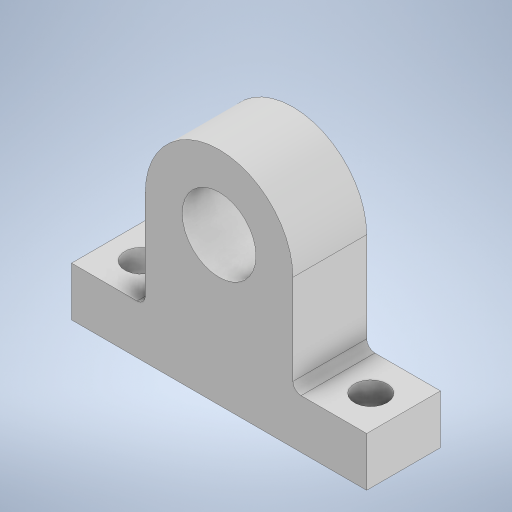
# Autodesk Inventor part: HUDSON 1-04-REAR DRAWBAR BEAM BRACKET
Saved by Autodesk Inventor 2024.2 (Build 282272000, 272)
## iProperties
Created: 2024-09-30
Part Number: HUDSON 1-04-REAR DRAWBAR BEAM BRACKET
Material: Generic
Document SubType Name: Modeling
Designer: Jimena Brenes
Density: 1 g/cm^3
Appearance: Default
Author: Jimena Brenes
Autodesk Inventor part; units mm, degrees
ref_plane "YZ Plane" through (0, 0, 0) normal (1, 0, 0) x (0, 1, 0)
ref_plane "XZ Plane" through (0, 0, 0) normal (0, 1, 0) x (-1, 0, 0)
ref_plane "XY Plane" through (0, 0, 0) normal (0, 0, 1) x (1, 0, 0)
sketch "Sketch1" plane through (0, 0, 0) normal (0, 0, 1) x (1, 0, 0)
  circle A0 centre (0, 0) radius 4.5
  arc A1 (9, 0) -> (-9, 0) centre (0, 0) ccw
  line L0 (0, 0) -> (0, -47) construction
  line L1 (0, -18) -> (-18, -18)
  line L2 (0, -18) -> (18, -18)
  line L3 (18, -18) -> (18, -12)
  line L4 (18, -12) -> (10, -12)
  line L5 (9, -11) -> (9, 0)
  line L6 (-18, -18) -> (-18, -12)
  line L7 (-18, -12) -> (-10, -12)
  line L8 (-9, -11) -> (-9, 0)
  arc A2 (-10, -12) -> (-9, -11) centre (-10, -11) ccw
  arc A3 (9, -11) -> (10, -12) centre (10, -11) ccw
  dimension "d0" = 9
  dimension "d1" = 18
  dimension "d6" = 6
  dimension "d7" = 6
  dimension "d9" = 18
  dimension "d10" = 2
  dimension "d11" = 2
  dimension "d12" = 9
  dimension "d13" = 9
  dimension "d14" = 36
  dimension "d15" = 18
  constraints: 18 end point, 6 point on circle, 5 perpendicular, 4 centre point, 4 tangent, 2 coincident, 2 horizontal, 2 vertical, 1 point on line
  measures "d0" diameter of A0
  measures "d1" diameter of A1
  measures "d6" distance between parallel lines of L2 L4
  measures "d7" distance of L1.end L6.end
  measures "d9" distance from line of L1 point (0, 0)
  measures "d10" diameter of A2
  measures "d11" diameter of A3
  measures "d12" distance from line of L8 L6.end
  measures "d13" distance from line of L5 L3.end
  measures "d14" distance between parallel lines of L3 L6
  measures "d15" distance of L1.start L2.end
extrude "Extrusion1" add sketch "Sketch1" against normal blind 9 contours A0 | L5 A3 L4 L3 L2 L1 L6 L7 A2 L8 A1
hole "Hole1" at (0, 0, 0) direction (0, 0, -1) diameter 9 end through all
sketch "Sketch2" plane through (-18, -12, 0) normal (0, 1, 0) x (1, 0, 0)
  circle A0 centre (4, 4.5) radius 2
  circle A1 centre (32, 4.5) radius 2
  line L0 (8, 0) -> (0, 0) projected
  line L1 (0, 0) -> (0, 9) projected
  line L2 (36, 0) -> (28, 0) projected
  line L3 (36, 0) -> (36, 9) projected
  point P0 (18, 0)
  dimension "d25" = 4
  dimension "d26" = 4
  dimension "d27" = 4.5
  dimension "d28" = 4
  dimension "d29" = 4.5
  dimension "d30" = 4
  constraints: 2 centre point
  measures "d25" diameter of A0
  measures "d26" diameter of A1
  measures "d27" distance from line of L0 A0.centre
  measures "d28" distance from line of L1 A0.centre
  measures "d29" distance from line of L2 A1.centre
  measures "d30" distance from line of L3 A1.centre
hole "Hole2" at (-14, -12, -4.5) at (14, -12, -4.5) direction (0, -1, 0) diameter 4 end through all
body "Solid1"
